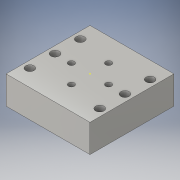
# Autodesk Inventor part: goniometer_stage_standoff_v01
Saved by Autodesk Inventor 2016 (Build 200138000, 138)
## iProperties
Created: 2017-01-09
Part Number: goniometer_stage_standoff_v01
Material: Stainless Steel AISI 304
Document SubType Name: Modeling
Designer: stephenholtz
Density: 8 g/cm^3
Appearance: Chrome - Satin
Author: stephenholtz
Autodesk Inventor part; units mm, degrees
ref_plane "YZ Plane" through (0, 0, 0) normal (1, 0, 0) x (0, 1, 0)
ref_plane "XZ Plane" through (0, 0, 0) normal (0, 1, 0) x (-1, 0, 0)
ref_plane "XY Plane" through (0, 0, 0) normal (0, 0, 1) x (1, 0, 0)
sketch "Sketch1" plane through (0, 0, 0) normal (0, 0, 1) x (1, 0, 0)
  line L0 (19.05, -19.05) -> (-19.05, -19.05)
  line L1 (-19.05, -19.05) -> (-19.05, 19.05)
  line L2 (-19.05, 19.05) -> (19.05, 19.05)
  line L3 (19.05, 19.05) -> (19.05, -19.05)
  line L4 (19.05, -19.05) -> (-19.05, 19.05) construction
  line L5 (-19.05, -19.05) -> (19.05, 19.05) construction
  point P0 (0, 0)
  dimension "d0" = 38.1
  dimension "d1" = 38.1
  constraints: 12 end point, 2 midpoint, 2 parallel, 1 horizontal, 1 perpendicular
  measures "d0" distance of L1.end L2.end
  measures "d1" distance of L0.end L1.end
extrude "Extrusion1" add sketch "Sketch1" along normal blind 12.7
sketch "Sketch4" plane through (0, 0, 12.7) normal (0, 0, 1) x (1, 0, 0)
  point P0 (0, 0)
sketch "Sketch5" plane through (0, 0, 12.7) normal (0, 0, 1) x (1, 0, 0)
  line L0 (-19.05, -19.05) -> (19.05, -19.05) construction
  line L1 (19.05, -19.05) -> (19.05, 19.05) construction
  line L2 (19.05, 19.05) -> (-19.05, 19.05) construction
  line L3 (-19.05, 19.05) -> (-19.05, -19.05) construction
  line L4 (15.875, -11.43) -> (-15.875, -11.43) construction
  line L5 (-15.875, -11.43) -> (-15.875, 11.43) construction
  line L6 (-15.875, 11.43) -> (15.875, 11.43) construction
  line L7 (15.875, 11.43) -> (15.875, -11.43) construction
  line L8 (15.875, -11.43) -> (-15.875, 11.43) construction
  line L9 (-15.875, -11.43) -> (15.875, 11.43) construction
  line L10 (11.43, -15.875) -> (-11.43, -15.875) construction
  line L11 (-11.43, -15.875) -> (-11.43, 15.875) construction
  line L12 (-11.43, 15.875) -> (11.43, 15.875) construction
  line L13 (11.43, 15.875) -> (11.43, -15.875) construction
  line L14 (11.43, -15.875) -> (-11.43, 15.875) construction
  line L15 (-11.43, -15.875) -> (11.43, 15.875) construction
  line L16 (0, -8.4414) -> (8.4414, 0) construction
  line L17 (8.4414, 0) -> (0, 8.4414) construction
  line L18 (0, 8.4414) -> (-8.4414, 0) construction
  line L19 (-8.4414, 0) -> (0, -8.4414) construction
  line L20 (-5.969, -5.969) -> (5.969, 5.969) construction
  line L21 (5.969, -5.969) -> (-5.969, 5.969) construction
  line L22 (-8.4414, -8.4414) -> (8.4414, -8.4414) construction
  line L23 (8.4414, -8.4414) -> (8.4414, 8.4414) construction
  line L24 (8.4414, 8.4414) -> (-8.4414, 8.4414) construction
  line L25 (-8.4414, 8.4414) -> (-8.4414, -8.4414) construction
  line L26 (-8.4414, -8.4414) -> (8.4414, 8.4414) construction
  line L27 (8.4414, -8.4414) -> (-8.4414, 8.4414) construction
  point P0 (0, 0)
  point P1 (0, 8.4414)
  point P2 (8.4414, 0)
  point P3 (-15.875, 0)
  point P4 (15.875, 0)
  point P5 (-15.875, 0)
  point P6 (-15.875, 0)
  point P7 (15.875, 0)
  dimension "d46" = 31.75
  dimension "d47" = 22.86
  dimension "d48" = 22.86
  dimension "d49" = 31.75
  dimension "d50" = 11.938
  dimension "d51" = 11.938
  dimension "d52" = 16.8829
  dimension "d53" = 16.8829
  dimension "d54" = 4.445
  dimension "d55" = 7.4336
  dimension "d56" = 5.969
  dimension "d57" = 5.969
  dimension "d58" = 4.445
  dimension "d59" = 7.4336
  dimension "d60" = 9.906
  dimension "d61" = 9.906
  dimension "d62" = 21.844
  dimension "d63" = 21.844
  dimension "d64" = 3.175
  dimension "d65" = 3.175
  constraints: 48 end point, 12 coincident, 10 parallel, 4 midpoint, 4 perpendicular, 3 horizontal, 3 point on line
  measures "d46" distance of L6.start L6.end
  measures "d47" distance of L9.start L6.start
  measures "d48" distance of L12.start L12.end
  measures "d49" distance of L10.end L12.start
  measures "d50" distance of L18.end L18.start
  measures "d51" distance of L18.start L16.end
  measures "d52" distance between parallel lines of L22 L24
  measures "d53" distance between parallel lines of L25 L23
  measures "d54" distance between parallel lines of L7 L13
  measures "d55" distance between parallel lines of L7 L23
  measures "d56" distance between parallel lines of L21 L17
  measures "d57" distance between parallel lines of L20 L16
  measures "d58" distance between parallel lines of L6 L12
  measures "d59" distance between parallel lines of L12 L24
  measures "d60" distance from line of L20.end L7
  measures "d61" distance from line of L21.start L7
  measures "d62" distance from line of L21.end L7
  measures "d63" distance from line of L20.start L7
  measures "d64" distance between parallel lines of L2 L12
  measures "d65" distance between parallel lines of L1 L7
hole "Hole2" at (-15.875, -11.43, 12.7) at (15.875, -11.43, 12.7) at (15.875, 0, 12.7) at (-15.875, 0, 12.7) at (-15.875, 11.43, 12.7) at (15.875, 11.43, 12.7) direction (0, 0, -1) diameter 3.7973 end through all
sketch "Sketch6" plane through (0, 0, 12.7) normal (0, 0, 1) x (1, 0, 0)
  circle A0 centre (-15.875, 11.43) radius 1.8986 construction
  circle A1 centre (15.875, 0) radius 1.8986 construction
  circle A2 centre (-15.875, -11.43) radius 1.8986 construction
  circle A3 centre (15.875, -11.43) radius 1.8986 construction
  circle A4 centre (-15.875, 0) radius 1.8986 construction
  circle A5 centre (15.875, 11.43) radius 1.8986 construction
  line L0 (-19.05, -19.05) -> (19.05, -19.05) construction
  line L1 (19.05, -19.05) -> (19.05, 19.05) construction
  line L2 (19.05, 19.05) -> (-19.05, 19.05) construction
  line L3 (-19.05, 19.05) -> (-19.05, -19.05) construction
  line L4 (15.875, -11.43) -> (-15.875, -11.43) construction
  line L5 (-15.875, -11.43) -> (-15.875, 11.43) construction
  line L6 (-15.875, 11.43) -> (15.875, 11.43) construction
  line L7 (15.875, 11.43) -> (15.875, -11.43) construction
  line L8 (15.875, -11.43) -> (-15.875, 11.43) construction
  line L9 (-15.875, -11.43) -> (15.875, 11.43) construction
  line L10 (11.43, -15.875) -> (-11.43, -15.875) construction
  line L11 (-11.43, -15.875) -> (-11.43, 15.875) construction
  line L12 (-11.43, 15.875) -> (11.43, 15.875) construction
  line L13 (11.43, 15.875) -> (11.43, -15.875) construction
  line L14 (11.43, -15.875) -> (-11.43, 15.875) construction
  line L15 (-11.43, -15.875) -> (11.43, 15.875) construction
  line L16 (0, -8.4414) -> (8.4414, 0) construction
  line L17 (8.4414, 0) -> (0, 8.4414) construction
  line L18 (0, 8.4414) -> (-8.4414, 0) construction
  line L19 (-8.4414, 0) -> (0, -8.4414) construction
  line L20 (-5.969, -5.969) -> (5.969, 5.969) construction
  line L21 (5.969, -5.969) -> (-5.969, 5.969) construction
  line L22 (-8.4414, -8.4414) -> (8.4414, -8.4414) construction
  line L23 (8.4414, -8.4414) -> (8.4414, 8.4414) construction
  line L24 (8.4414, 8.4414) -> (-8.4414, 8.4414) construction
  line L25 (-8.4414, 8.4414) -> (-8.4414, -8.4414) construction
  line L26 (-8.4414, -8.4414) -> (8.4414, 8.4414) construction
  line L27 (8.4414, -8.4414) -> (-8.4414, 8.4414) construction
  point P0 (0, 0)
  point P1 (0, 8.4414)
  point P2 (8.4414, 0)
  point P3 (8.4414, 0)
  dimension "d73" = 31.75
  dimension "d74" = 22.86
  dimension "d75" = 22.86
  dimension "d76" = 31.75
  dimension "d77" = 11.938
  dimension "d78" = 11.938
  dimension "d79" = 16.8829
  dimension "d80" = 16.8829
  dimension "d81" = 4.445
  dimension "d82" = 7.4336
  dimension "d83" = 5.969
  dimension "d84" = 5.969
  dimension "d85" = 4.445
  dimension "d86" = 7.4336
  dimension "d87" = 9.906
  dimension "d88" = 9.906
  dimension "d89" = 21.844
  dimension "d90" = 21.844
  dimension "d91" = 3.175
  dimension "d92" = 3.175
  constraints: 48 end point, 10 parallel, 4 coincident, 4 perpendicular, 3 horizontal, 3 point on line, 2 midpoint
  measures "d73" distance of L6.start L6.end
  measures "d74" distance of L5.start L6.start
  measures "d75" distance of L11.end L15.end
  measures "d76" distance of L11.start L11.end
  measures "d77" distance of L18.end L17.end
  measures "d78" distance of L17.end L17.start
  measures "d79" distance between parallel lines of L22 L24
  measures "d80" distance between parallel lines of L25 L23
  measures "d81" distance between parallel lines of L7 L13
  measures "d82" distance between parallel lines of L7 L23
  measures "d83" distance between parallel lines of L21 L17
  measures "d84" distance between parallel lines of L20 L16
  measures "d85" distance between parallel lines of L6 L12
  measures "d86" distance between parallel lines of L12 L24
  measures "d87" distance from line of L20.end L7
  measures "d88" distance from line of L21.start L7
  measures "d89" distance from line of L21.end L7
  measures "d90" distance from line of L20.start L7
  measures "d91" distance between parallel lines of L2 L12
  measures "d92" distance between parallel lines of L1 L7
hole "Hole3" at (-8.4414, 0, 12.7) at (0, 8.4414, 12.7) at (8.4414, 0, 12.7) at (0, -8.4414, 12.7) direction (0, 0, -1) diameter 2.7051 depth 6.35 tip angle 118
body "Solid1"
